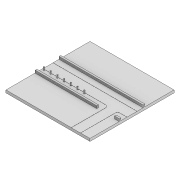
# Autodesk Inventor part: scene2
Saved by Autodesk Inventor 2021 (Build 250183000, 183)
## iProperties
Created: 2022-03-08
Part Number: scene2
Material: Generic
Document SubType Name: Modeling
Designer: Derm
Density: 1 g/cm^3
Appearance: Default
Author: Derm
Autodesk Inventor part; units mm, degrees
ref_plane "YZ Plane" through (0, 0, 0) normal (1, 0, 0) x (0, 1, 0)
ref_plane "XZ Plane" through (0, 0, 0) normal (0, 1, 0) x (-1, 0, 0)
ref_plane "XY Plane" through (0, 0, 0) normal (0, 0, 1) x (1, 0, 0)
sketch "Sketch1" plane through (0, 0, 0) normal (0, 1, 0) x (-1, 0, 0)
  line L0 (50000, 50000) -> (-50000, 50000)
  line L1 (-50000, 50000) -> (-50000, -50000)
  line L2 (-50000, -50000) -> (50000, -50000)
  line L3 (50000, -50000) -> (50000, 50000)
  line L4 (50000, 50000) -> (-50000, -50000) construction
  line L5 (-50000, 50000) -> (50000, -50000) construction
  point P0 (0, 0)
  dimension "d0" = 100000
  dimension "d1" = 100000
  constraints: 12 end point, 2 midpoint, 2 parallel, 1 horizontal, 1 perpendicular
  measures "d0" distance of L1.end L2.end
  measures "d1" distance of L0.end L1.end
extrude "Extrusion1" add sketch "Sketch1" against normal blind 3000
sketch "Sketch2" plane through (0, 0, 0) normal (0, 1, 0) x (1, 0, 0)
  line L0 (50000, -50000) -> (50000, 50000) projected
  line L1 (50000, 50000) -> (-50000, 50000) projected
  line L2 (-50000, 50000) -> (-50000, -50000) projected
  line L3 (-50000, -50000) -> (50000, -50000) projected
  line L4 (50000, 50000) -> (50000, -50000) projected
  line L5 (-50000, -6000) -> (50000, -6000)
  line L6 (50000, -6000) -> (50000, 6000)
  line L7 (-50000, 6000) -> (-50000, -6000)
  line L8 (-50000, -6000) -> (50000, 6000) construction
  line L9 (50000, -6000) -> (-50000, 6000) construction
  line L10 (-50000, 50000) -> (50000, 50000) projected
  line L11 (38735.1966, 9000) -> (38735.1966, 50000)
  line L12 (38735.1966, 50000) -> (27735.1966, 50000)
  line L13 (27735.1966, 50000) -> (27735.1966, 9000)
  line L14 (50000, 6000) -> (41735.1966, 6000)
  line L15 (24735.1966, 6000) -> (-50000, 6000)
  arc A0 (24735.1966, 6000) -> (27735.1966, 9000) centre (24735.1966, 9000) ccw
  arc A1 (38735.1966, 9000) -> (41735.1966, 6000) centre (41735.1966, 9000) ccw
  point P0 (0, 0)
  dimension "d5" = 11000
  dimension "d6" = 3000
  constraints: 20 end point, 4 parallel, 4 point on circle, 4 tangent, 2 centre point, 2 midpoint, 2 point on line, 1 equal radius, 1 horizontal, 1 perpendicular
  measures "d5" distance between parallel lines of L11 L13
  measures "d6" radius of A0
extrude "Extrusion2" cut sketch "Sketch2" against normal blind 100 contours L5 L2 L15 A0 L13 L1 L11 A1 L14 L0
sketch "Sketch3" plane through (0, 0, 0) normal (0, 1, 0) x (1, 0, 0)
  line L0 (50000, 50000) -> (50000, -50000) projected
  line L1 (50000, -50000) -> (-50000, -50000) projected
  line L2 (-50000, -50000) -> (-50000, 50000) projected
  line L3 (-50000, 50000) -> (50000, 50000) projected
  line L4 (-50000, 6000) -> (24735.1966, 6000) projected
  arc A0 (24735.1966, 6000) -> (27735.1966, 9000) centre (24735.1966, 9000) ccw projected
  line L5 (27735.1966, 9000) -> (27735.1966, 50000) projected
  line L6 (27735.1966, 50000) -> (-50000, 50000) projected
  line L7 (-50000, 50000) -> (-50000, 6000) projected
  line L8 (23068.1077, 10876.2035) -> (6908.7226, 10876.2035)
  line L9 (6908.7226, 10876.2035) -> (6908.7226, 28000)
  line L10 (6908.7226, 28000) -> (23068.1077, 28000)
  line L11 (23068.1077, 28000) -> (23068.1077, 10876.2035)
  line L12 (23068.1077, 10876.2035) -> (6908.7226, 28000) construction
  line L13 (6908.7226, 10876.2035) -> (23068.1077, 28000) construction
  point P0 (0, 0)
  point P1 (14988.4151, 19438.1018)
  constraints: 12 end point, 2 midpoint, 2 parallel, 1 horizontal, 1 perpendicular
extrude "Extrusion3" add sketch "Sketch3" along normal blind 5000 contours L8 L9 L10 L11
sketch "Sketch4" plane through (23068.1077, 0, -28000) normal (0, 0, -1) x (-1, 0, 0)
  line L0 (16159.3851, 0) -> (0, 0) projected
  line L1 (16159.3851, 0) -> (16159.3851, 5000) projected
  line L2 (0, 5000) -> (16159.3851, 5000) projected
  line L3 (0, 0) -> (0, 5000) projected
  line L4 (0, 5000) -> (16159.3851, 5000) projected
  line L5 (0, 5000) -> (-502.206, 5000)
  line L6 (-502.206, 5000) -> (1674.3292, 8799.2208)
  line L7 (1674.3292, 8799.2208) -> (8079.6925, 8799.2208)
  line L8 (8079.6925, 5000) -> (8079.6925, 8799.2208)
  line L9 (16159.3851, 5000) -> (16661.5911, 5000)
  line L10 (16661.5911, 5000) -> (14485.0559, 8799.2208)
  line L11 (14485.0559, 8799.2208) -> (8079.6925, 8799.2208)
  point P0 (23068.1077, 0)
  constraints: 14 end point, 2 symmetric about line, 1 horizontal, 1 midpoint, 1 parallel, 1 perpendicular
extrude "Extrusion4" add sketch "Sketch4" against normal up to surface (17123.7965 mm away) contours L2 L8 L11 L10 L9 | L5 L6 L7 L8 L2
sketch "Sketch5" plane through (6908.7226, 0, -10876.2035) normal (0, 0, 1) x (1, 0, 0)
  line L0 (16159.3851, 0) -> (0, 0) projected
  line L1 (16159.3851, 0) -> (16159.3851, 5000) projected
  line L2 (16661.5911, 5000) -> (16159.3851, 5000) projected
  line L3 (14485.0559, 8799.2208) -> (16661.5911, 5000) projected
  line L4 (1674.3292, 8799.2208) -> (14485.0559, 8799.2208) projected
  line L5 (-502.206, 5000) -> (1674.3292, 8799.2208) projected
  line L6 (0, 5000) -> (-502.206, 5000) projected
  line L7 (0, 0) -> (0, 5000) projected
  line L8 (0, 5000) -> (-502.206, 5000) projected
  line L9 (16661.5911, 5000) -> (16159.3851, 5000) projected
  line L10 (0, 5000) -> (16159.3851, 5000)
  point P0 (-6908.7226, 0)
  constraints: 2 end point, 1 collinear
extrude "Extrusion5" add sketch "Sketch5" along normal blind 600 contours L10 L6 L5 L4 L3 L2
ref_plane "Work Plane1" through (23068.1077, 0, -19438.1018) normal (0, 0, -1) x (-1, 0, 0)
mirror "Mirror1" about plane through (23068.1077, 0, -19438.1018) normal (0, 0, -1) of "Extrusion5"
chamfer "Chamfer1" distance 50 angle 45 7 edges at (-12632.4017, 0, -6000) (26856.517, 0, -6878.6797) (27735.1966, 0, -29500) (0, 0, 6000) (38735.1966, 0, -29500) (39613.8763, 0, -6878.6797) (45867.5983, 0, -6000)
chamfer "Chamfer2" distance 3500 angle 45 2 edges at (14988.4151, 8799.2208, -10276.2035) (14988.4151, 8799.2208, -28600)
sketch "Sketch6" plane through (0, 0, 0) normal (0, 1, 0) x (1, 0, 0)
  line L0 (-50000, -6050) -> (50000, -6050) projected
  line L1 (-50000, -6050) -> (-50000, -50000) projected
  line L2 (-50000, -50000) -> (50000, -50000) projected
  line L3 (50000, -50000) -> (50000, -6050) projected
  circle A0 centre (0, -6758.2768) radius 750
  point P0 (0, 0)
  dimension "d21" = 1500
  constraints: 1 centre point
  measures "d21" diameter of A0
extrude "Extrusion6" add sketch "Sketch6" along normal blind 3000 contours A0 L0 | L0 A0
pattern_linear "Rectangular Pattern1" count 7 spacing 8000 along (-1, 0, 0) of "Extrusion6"
sketch "Sketch7" plane through (0, 0, 0) normal (0, 1, 0) x (1, 0, 0)
  arc A0 (-40246.6658, -6050) -> (-39753.3342, -6050) centre (-40000, -6758.2768) ccw projected
  arc A1 (-24246.6658, -6050) -> (-23753.3342, -6050) centre (-24000, -6758.2768) ccw projected
  arc A2 (-8246.6658, -6050) -> (-7753.3342, -6050) centre (-8000, -6758.2768) ccw projected
  arc A3 (-16246.6658, -6050) -> (-15753.3342, -6050) centre (-16000, -6758.2768) ccw projected
  arc A4 (-32246.6658, -6050) -> (-31753.3342, -6050) centre (-32000, -6758.2768) ccw projected
  arc A5 (-246.6658, -6050) -> (246.6658, -6050) centre (0, -6758.2768) ccw projected
  line L0 (-50000, -6050) -> (-48246.6658, -6050) projected
  line L1 (-50000, -6050) -> (-50000, -50000) projected
  line L2 (-50000, -50000) -> (50000, -50000) projected
  line L3 (50000, -50000) -> (50000, -6050) projected
  line L4 (-50000, -6050) -> (-50000, -50000) projected
  line L5 (50000, 50000) -> (50000, -50000) projected
  line L6 (-50000, -15243.9206) -> (50000, -15243.9206)
  line L7 (50000, -15243.9206) -> (50000, -13182.5289)
  line L8 (50000, -13182.5289) -> (-50000, -13182.5289)
  line L9 (-50000, -13182.5289) -> (-50000, -15243.9206)
  arc A6 (-48246.6658, -6050) -> (-47753.3342, -6050) centre (-48000, -6758.2768) ccw projected
  line L10 (246.6658, -6050) -> (50000, -6050) projected
  line L11 (-7753.3342, -6050) -> (-246.6658, -6050) projected
  line L12 (-15753.3342, -6050) -> (-8246.6658, -6050) projected
  line L13 (-23753.3342, -6050) -> (-16246.6658, -6050) projected
  line L14 (-31753.3342, -6050) -> (-24246.6658, -6050) projected
  line L15 (-39753.3342, -6050) -> (-32246.6658, -6050) projected
  line L16 (-47753.3342, -6050) -> (-40246.6658, -6050) projected
  point P0 (0, 0)
  point P1 (-50000, -13182.5289)
  point P2 (50000, -15243.9206)
  constraints: 8 end point, 2 parallel, 2 point on line, 1 horizontal, 1 perpendicular
extrude "Extrusion7" add sketch "Sketch7" along normal blind 3000 contours L8 L3 L6 L1
sketch "Sketch8" plane through (0, 0, 0) normal (0, 0, 1) x (1, 0, 0)
  line L0 (-60036.3598, 14647.1686) -> (68892.7873, 14647.1686)
  line L1 (68892.7873, 14647.1686) -> (68892.7873, -8515.7957)
  line L2 (68892.7873, -8515.7957) -> (-60036.3598, -8515.7957)
  line L3 (-60036.3598, -8515.7957) -> (-60036.3598, 14647.1686)
  point P0 (0, 0)
  constraints: 8 end point, 2 parallel, 1 horizontal, 1 perpendicular
extrude "Extrusion8" cut sketch "Sketch8" against normal through all
mirror "Mirror2" about plane through (4428.2138, 3065.6864, 0) normal (0, 0, -1) of "Extrusion2", "Extrusion1", "Extrusion7"
sketch "Sketch9" plane through (-50000, -100, -6000) normal (0, 1, 0) x (1, 0, 0)
  line L0 (0, -12000) -> (74735.1966, -12000) projected
  arc A0 (77735.1966, -15000) -> (74735.1966, -12000) centre (74735.1966, -15000) ccw projected
  line L1 (77735.1966, -15000) -> (77735.1966, -56000) projected
  line L2 (88735.1966, -56000) -> (77735.1966, -56000) projected
  line L3 (88735.1966, -56000) -> (88735.1966, -15000) projected
  arc A1 (91735.1966, -12000) -> (88735.1966, -15000) centre (91735.1966, -15000) ccw projected
  line L4 (91735.1966, -12000) -> (100000, -12000) projected
  line L5 (100000, 0) -> (100000, -12000) projected
  line L6 (100000, 0) -> (0, 0) projected
  line L7 (0, -12000) -> (0, 0) projected
  arc A2 (77735.1966, -15000) -> (74735.1966, -12000) centre (74735.1966, -15000) ccw projected
  arc A3 (91735.1966, -12000) -> (88735.1966, -15000) centre (91735.1966, -15000) ccw projected
  line L8 (91735.1966, -12000) -> (74735.1966, -12000)
  point P0 (50000, -6000)
  constraints: 2 end point, 2 tangent, 1 horizontal
extrude "Extrusion9" [suppressed]
sketch "Sketch10" plane through (-50000, -100, 6000) normal (0, 1, 0) x (1, 0, 0)
  line L0 (91735.1966, 0) -> (100000, 0) projected
  line L1 (100000, 12000) -> (100000, 0) projected
  line L2 (100000, 12000) -> (0, 12000) projected
  line L3 (0, 0) -> (0, 12000) projected
  line L4 (0, 0) -> (74735.1966, 0) projected
  arc A0 (77735.1966, -3000) -> (74735.1966, 0) centre (74735.1966, -3000) ccw projected
  line L5 (77735.1966, -3000) -> (77735.1966, -44000) projected
  line L6 (88735.1966, -44000) -> (77735.1966, -44000) projected
  line L7 (88735.1966, -44000) -> (88735.1966, -3000) projected
  arc A1 (91735.1966, 0) -> (88735.1966, -3000) centre (91735.1966, -3000) ccw projected
  point P0 (50000, 6000)
extrude "Extrusion10" [suppressed]
sketch "Sketch11" plane through (0, 3000, 0) normal (0, 1, 0) x (1, 0, 0)
  line L0 (-50000, -13182.5289) -> (-50000, -15243.9206) projected
  line L1 (-50000, -15243.9206) -> (50000, -15243.9206) projected
  line L2 (50000, -15243.9206) -> (50000, -13182.5289) projected
  line L3 (50000, -13182.5289) -> (-50000, -13182.5289) projected
  line L4 (50000, -13182.5289) -> (-50000, -13182.5289) projected
  line L5 (-50000, -15243.9206) -> (50000, -15243.9206) projected
  line L6 (44357.964, -13182.5289) -> (23293.9294, -13182.5289)
  line L7 (23293.9294, -13182.5289) -> (23293.9294, -15243.9206)
  line L8 (23293.9294, -15243.9206) -> (44357.964, -15243.9206)
  line L9 (44357.964, -15243.9206) -> (44357.964, -13182.5289)
  point P0 (0, 0)
  point P1 (44357.964, -15243.9206)
  constraints: 8 end point, 2 parallel, 2 point on line, 1 horizontal, 1 perpendicular
extrude "Extrusion11" cut sketch "Sketch11" against normal up to surface (3000 mm away) contours L3 L9 L1 L7
sketch "Sketch12" plane through (0, 0, 0) normal (0, 1, 0) x (1, 0, 0)
  line L0 (24735.1966, -6000) -> (-50000, -6000) projected
  line L1 (-50000, -6000) -> (-50000, -13182.5289) projected
  line L2 (-50000, -13182.5289) -> (23293.9294, -13182.5289) projected
  line L3 (23293.9294, -15243.9206) -> (23293.9294, -13182.5289) projected
  line L4 (23293.9294, -15243.9206) -> (-50000, -15243.9206) projected
  line L5 (-50000, -15243.9206) -> (-50000, -50000) projected
  line L6 (-50000, -50000) -> (27735.1966, -50000) projected
  line L7 (27735.1966, -50000) -> (27735.1966, -9000) projected
  arc A0 (27735.1966, -9000) -> (24735.1966, -6000) centre (24735.1966, -9000) ccw projected
  circle A1 centre (-48000, -6758.2768) radius 750 projected
  circle A2 centre (-40000, -6758.2768) radius 750 projected
  circle A3 centre (-32000, -6758.2768) radius 750 projected
  circle A4 centre (-24000, -6758.2768) radius 750 projected
  circle A5 centre (-16000, -6758.2768) radius 750 projected
  circle A6 centre (-8000, -6758.2768) radius 750 projected
  circle A7 centre (0, -6758.2768) radius 750 projected
  line L8 (-50000, 15243.9206) -> (50000, 15243.9206) projected
  line L9 (50000, 15243.9206) -> (50000, 50000) projected
  line L10 (-50000, 50000) -> (50000, 50000) projected
  line L11 (-50000, 50000) -> (-50000, 15243.9206) projected
  line L12 (50000, 13182.5289) -> (-50000, 13182.5289) projected
  line L13 (-50000, 13182.5289) -> (-50000, 6000) projected
  line L14 (-50000, 6000) -> (50000, 6000) projected
  line L15 (50000, 6000) -> (50000, 13182.5289) projected
  line L16 (50000, -6000) -> (41735.1966, -6000) projected
  arc A8 (41735.1966, -6000) -> (38735.1966, -9000) centre (41735.1966, -9000) ccw projected
  line L17 (38735.1966, -9000) -> (38735.1966, -50000) projected
  line L18 (38735.1966, -50000) -> (50000, -50000) projected
  line L19 (50000, -50000) -> (50000, -15243.9206) projected
  line L20 (50000, -15243.9206) -> (44357.964, -15243.9206) projected
  line L21 (44357.964, -13182.5289) -> (44357.964, -15243.9206) projected
  line L22 (44357.964, -13182.5289) -> (50000, -13182.5289) projected
  line L23 (50000, -13182.5289) -> (50000, -6000) projected
  point P0 (0, 0)
extrude "Extrusion12" add sketch "Sketch12" along normal blind 100
sketch "Sketch13" plane through (-50000, -100, -6000) normal (0, 1, 0) x (1, 0, 0)
  line L0 (0, -12000) -> (74735.1966, -12000) projected
  arc A0 (77735.1966, -15000) -> (74735.1966, -12000) centre (74735.1966, -15000) ccw projected
  line L1 (77735.1966, -15000) -> (77735.1966, -56000) projected
  line L2 (88735.1966, -56000) -> (77735.1966, -56000) projected
  line L3 (88735.1966, -56000) -> (88735.1966, -15000) projected
  arc A1 (91735.1966, -12000) -> (88735.1966, -15000) centre (91735.1966, -15000) ccw projected
  line L4 (91735.1966, -12000) -> (100000, -12000) projected
  line L5 (100000, 0) -> (100000, -12000) projected
  line L6 (100000, 0) -> (0, 0) projected
  line L7 (0, -12000) -> (0, 0) projected
  point P0 (50000, -6000)
extrude "Extrusion13" add sketch "Sketch13" along normal blind 100
body "Solid1"
